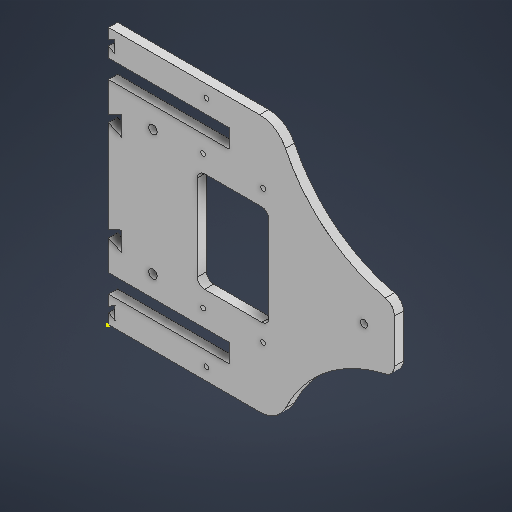
# Autodesk Inventor part: amir
Saved by Autodesk Inventor 2026.1 (Build 301233020, 233B)
## iProperties
Created: 2026-01-26
Part Number: amir
Material: Genérico
Document SubType Name: Modeling
Designer: i5
Density: 1 g/cm^3
Appearance: Valor por defecto
Author: i5
Autodesk Inventor part; units mm, degrees
ref_plane "YZ Plane" through (0, 0, 0) normal (1, 0, 0) x (0, 1, 0)
ref_plane "XZ Plane" through (0, 0, 0) normal (0, 1, 0) x (-1, 0, 0)
ref_plane "XY Plane" through (0, 0, 0) normal (0, 0, 1) x (1, 0, 0)
sketch "Boceto1" plane through (0, 0, 0) normal (0, 0, 1) x (1, 0, 0)
  line L0 (0.0213, 161.5) -> (84.4213, 161.5)
  line L1 (0.0213, 180) -> (0.0213, 172.7)
  line L2 (0.0213, 161.5) -> (0.0213, 168.8)
  line L3 (4.5413, 170.75) -> (4.5413, 175.3)
  line L4 (4.5413, 175.3) -> (0.0213, 172.7)
  line L5 (4.5413, 170.75) -> (4.5413, 166.2)
  line L6 (4.5413, 166.2) -> (0.0213, 168.8)
  line L7 (0.0213, 161.5) -> (84.4213, 161.5)
  line L8 (84.4213, 161.5) -> (84.4213, 148.5)
  line L9 (84.4213, 148.5) -> (0.0213, 148.5)
  line L10 (0.0213, 148.5) -> (0.0213, 127.5)
  line L11 (9.1213, 124.95) -> (9.1213, 131.75)
  line L12 (9.1213, 131.75) -> (0.0213, 127.5)
  line L13 (9.1213, 124.95) -> (9.1213, 118.15)
  line L14 (9.1213, 118.15) -> (0.0213, 122.4)
  line L15 (0.0213, 122.4) -> (0.0213, 90)
  line L16 (0.0213, 180) -> (105.7213, 180)
  line L17 (200.0213, 90) -> (200.0213, 105.2)
  arc A0 (200.0213, 105.2) -> (193.7585, 113.0091) centre (192.0213, 105.2) ccw
  arc A1 (123.7591, 168.6393) -> (105.7213, 180) centre (105.7213, 160) ccw
  arc A2 (123.7591, 168.6393) -> (193.7585, 113.0091) centre (215.9584, 212.7984) ccw
  line L18 (62.2213, 90) -> (62.2213, 120)
  line L19 (112.2213, 120) -> (112.2213, 90)
  circle A3 centre (178.7213, 90) radius 2.5
  circle A4 centre (31.1213, 133.75) radius 3
  line L20 (67.2213, 125) -> (87.2213, 125)
  arc A5 (67.2213, 125) -> (62.2213, 120) centre (67.2213, 120) ccw
  circle A6 centre (66.2213, 136.75) radius 1.65
  circle A7 centre (108.2213, 136.75) radius 1.65
  circle A8 centre (68.5213, 171.35) radius 1.65
  line L21 (87.2213, 125) -> (107.2213, 125)
  arc A9 (112.2213, 120) -> (107.2213, 125) centre (107.2213, 120) ccw
  line L22 (0.0213, 18.5) -> (84.4213, 18.5)
  line L23 (0.0213, 0) -> (0.0213, 7.3)
  line L24 (0.0213, 18.5) -> (0.0213, 11.2)
  line L25 (4.5413, 9.25) -> (4.5413, 4.7)
  line L26 (4.5413, 4.7) -> (0.0213, 7.3)
  line L27 (4.5413, 9.25) -> (4.5413, 13.8)
  line L28 (4.5413, 13.8) -> (0.0213, 11.2)
  line L29 (0.0213, 18.5) -> (84.4213, 18.5)
  line L30 (84.4213, 18.5) -> (84.4213, 31.5)
  line L31 (84.4213, 31.5) -> (0.0213, 31.5)
  line L32 (0.0213, 31.5) -> (0.0213, 52.5)
  line L33 (9.1213, 55.05) -> (9.1213, 48.25)
  line L34 (9.1213, 48.25) -> (0.0213, 52.5)
  line L35 (9.1213, 55.05) -> (9.1213, 61.85)
  line L36 (9.1213, 61.85) -> (0.0213, 57.6)
  line L37 (0.0213, 57.6) -> (0.0213, 90)
  line L38 (0.0213, 0) -> (105.7213, 0)
  line L39 (200.0213, 90) -> (200.0213, 74.8)
  arc A10 (193.7585, 66.9909) -> (200.0213, 74.8) centre (192.0213, 74.8) ccw
  arc A11 (105.7213, 0) -> (123.7591, 11.3607) centre (105.7213, 20) ccw
  arc A12 (193.7585, 66.9909) -> (123.7591, 11.3607) centre (215.9584, -32.7984) ccw
  line L40 (62.2213, 90) -> (62.2213, 60)
  line L41 (112.2213, 60) -> (112.2213, 90)
  circle A13 centre (178.7213, 90) radius 2.5
  circle A14 centre (31.1213, 46.25) radius 3
  line L42 (67.2213, 55) -> (87.2213, 55)
  arc A15 (62.2213, 60) -> (67.2213, 55) centre (67.2213, 60) ccw
  circle A16 centre (66.2213, 43.25) radius 1.65
  circle A17 centre (108.2213, 43.25) radius 1.65
  circle A18 centre (68.5213, 8.65) radius 1.65
  line L43 (87.2213, 55) -> (107.2213, 55)
  arc A19 (107.2213, 55) -> (112.2213, 60) centre (107.2213, 60) ccw
  point P0 (0, 0)
  constraints: 88 end point, 20 centre point, 20 point on circle
extrude "Extrusión1" add sketch "Boceto1" along normal blind 6.35
fillet "Empalme1" radius 0.01 26 edges at (116.38, 176.9231, 0) (152.3544, 132.7655, 0) (198.2622, 110.2051, 0) (200.0213, 97.6, 0) (198.2622, 69.7949, 0) (152.3544, 47.2345, 0) (116.38, 3.0769, 0) (52.8713, 0, 0) (52.8713, 180, 0) (116.38, 176.9231, 6.35) (152.3544, 132.7655, 6.35) (198.2622, 110.2051, 6.35) (200.0213, 97.6, 6.35) (198.2622, 69.7949, 6.35) (152.3544, 47.2345, 6.35) (116.38, 3.0769, 6.35) (52.8713, 0, 6.35) (52.8713, 180, 6.35) (0.0213, 180, 3.175) (0.0213, 138, 6.35) (0.0213, 138, 0) (0.0213, 106.2, 6.35) (0.0213, 106.2, 0) (0.0213, 42, 6.35) (0.0213, 42, 0) (4.5413, 6.975, 0)
sketch "Boceto2" plane through (0, 0, 6.35) normal (0, 0, 1) x (1, 0, 0)
  point P0 (0, 0)
